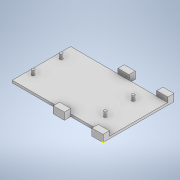
# Autodesk Inventor part: b
Saved by Autodesk Inventor 2021 (Build 250183000, 183)
## iProperties
Created: 2020-05-22
Part Number: b
Material: Generic
Document SubType Name: Modeling
Designer: andre
Density: 1 g/cm^3
Appearance: Default
Author: andre
Autodesk Inventor part; units mm, degrees
ref_plane "YZ Plane" through (0, 0, 0) normal (1, 0, 0) x (0, 1, 0)
ref_plane "XZ Plane" through (0, 0, 0) normal (0, 1, 0) x (-1, 0, 0)
ref_plane "XY Plane" through (0, 0, 0) normal (0, 0, 1) x (1, 0, 0)
sketch "Sketch1" plane through (0, 0, 0) normal (0, 1, 0) x (-1, 0, 0)
  line L0 (0, 0) -> (7, 0)
  line L1 (7, 0) -> (7, -4)
  line L2 (7, -4) -> (0, -4)
  line L3 (0, -4) -> (0, 0)
  line L4 (0, -22.5) -> (26.9418, -22.5) construction
  line L5 (24.5, 0) -> (31.5, 0)
  line L6 (31.5, 0) -> (31.5, -4)
  line L7 (31.5, -4) -> (24.5, -4)
  line L8 (24.5, -4) -> (24.5, 0)
  line L9 (0, -45) -> (7, -45)
  line L10 (7, -45) -> (7, -41)
  line L11 (7, -41) -> (0, -41)
  line L12 (0, -41) -> (0, -45)
  line L13 (24.5, -45) -> (31.5, -45)
  line L14 (31.5, -45) -> (31.5, -41)
  line L15 (31.5, -41) -> (24.5, -41)
  line L16 (24.5, -41) -> (24.5, -45)
  dimension "d0" = 7
  dimension "d1" = 4
  dimension "d2" = 18.5
  dimension "d3" = 7
  dimension "d4" = 17.5
  dimension "d5" = 37
  dimension "d15" = 4
  constraints: 34 end point, 8 symmetric about line, 4 parallel, 3 horizontal, 2 perpendicular
  measures "d0" distance of L0.start L0.end
  measures "d1" distance of L2.end L0.start
  measures "d2" distance between parallel lines of L4 L2
  measures "d3" distance of L5.start L5.end
  measures "d4" distance between parallel lines of L1 L8
  measures "d5" distance between parallel lines of L11 L2
  measures "d15" distance between parallel lines of L15 L13
extrude "Extrusion1" add sketch "Sketch1" along normal blind 4.5
sketch "Sketch2" plane through (0, 0, -4) normal (0, 0, -1) x (-1, 0, 0)
  line L0 (0, 0) -> (7, 0) projected
  line L1 (31.5, 0) -> (31.5, 4.5) projected
  line L2 (0, 0) -> (31.5, 0)
  line L3 (31.5, 0) -> (31.5, 1.5)
  line L4 (31.5, 1.5) -> (0, 1.5)
  line L5 (0, 1.5) -> (0, 0)
  dimension "d8" = 1.5
  dimension "d11" = 31.5
  constraints: 8 end point, 2 parallel, 1 horizontal, 1 perpendicular, 1 point on line
  measures "d8" distance of L3.end L2.end
  measures "d11" distance of L0.start L2.end
extrude "Extrusion2" add sketch "Sketch2" along normal blind 37
sketch "Sketch3" plane through (0, 0, 0) normal (0, -1, 0) x (1, 0, 0)
  point P0 (0, 0)
sketch "Sketch4" plane through (-31.5, 0, 0) normal (-1, 0, 0) x (0, 0, 1)
  line L0 (-41, 1.5) -> (-41, 4.5) projected
  line L1 (0, 0) -> (-45, 0) projected
  line L2 (-41, 1.5) -> (-4, 1.5)
  line L3 (-4, 1.5) -> (-4, 0)
  line L4 (-4, 0) -> (-41, 0)
  line L5 (-41, 0) -> (-41, 1.5)
  point P0 (-41, 0)
  dimension "d12" = 37
  constraints: 8 end point, 2 parallel, 1 horizontal, 1 perpendicular, 1 point on line
  measures "d12" distance of L3.end L4.end
extrude "Extrusion3" add sketch "Sketch4" along normal blind 30
sketch "Sketch5" plane through (-24.5, 1.5, -4) normal (0, 1, 0) x (1, 0, 0)
  circle A0 centre (12.2952, 27.39) radius 0.9
  line L0 (24.5, -4) -> (24.5, 41) construction
  line L1 (24.5, 18.5) -> (-15.4775, 18.5) construction
  circle A1 centre (-33.4248, 27.39) radius 0.9
  circle A2 centre (12.2952, 9.61) radius 0.9
  circle A3 centre (-33.4248, 9.61) radius 0.9
  dimension "d16" = 1.8
  dimension "d17" = 8.89
  dimension "d18" = 1.8
  dimension "d19" = 45.72
  dimension "d22" = 8.89
  constraints: 4 centre point, 2 end point, 2 symmetric about line, 1 horizontal, 1 midpoint, 2 other
  measures "d16" diameter of A0
  measures "d17" distance from line of L1 A0.centre
  measures "d18" diameter of A1
  measures "d19" distance of A1.centre A0.centre
  measures "d22" distance from line of L1 A1.centre
extrude "Extrusion4" add sketch "Sketch5" along normal blind 3
equation "\"d3\" = d0"
equation "\"d18\" = d16"
equation "\"d22\" = d17"
body "Solid1"
